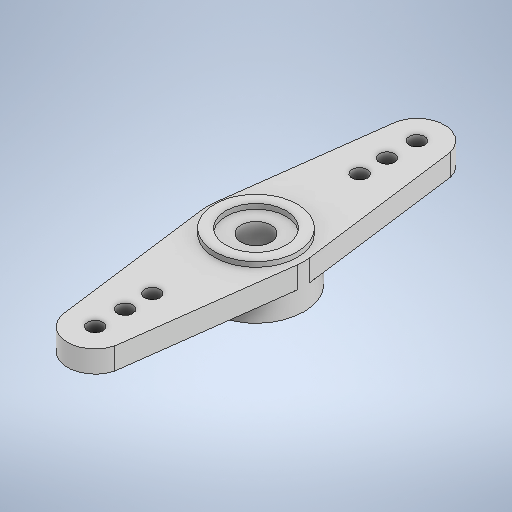
# Autodesk Inventor part: MMAE 232 Assignment 2_White Propellor - Dylan Tamras
Saved by Autodesk Inventor 2025.2 (Build 292293000, 293)
## iProperties
Created: 2025-01-19
Part Number: MMAE 232 Assignment 2_White Propellor - Dylan Tamras
Material: Generic
Document SubType Name: Modeling
Designer: Dylan
Density: 1 g/cm^3
Appearance: Default
Author: VRK99-0110
Title: Servo - White Propellor
Autodesk Inventor part; units mm, degrees
ref_plane "YZ Plane" through (0, 0, 0) normal (1, 0, 0) x (0, 1, 0)
ref_plane "XZ Plane" through (0, 0, 0) normal (0, 1, 0) x (-1, 0, 0)
ref_plane "XY Plane" through (0, 0, 0) normal (0, 0, 1) x (1, 0, 0)
sketch "Sketch1" plane through (0, 0, 0) normal (0, 1, 0) x (-1, 0, 0)
  line L0 (0, 0) -> (0, -14.74)
  arc A0 (-2.52, -14.74) -> (2.52, -14.74) centre (0, -14.74) ccw
  line L1 (2.4362, -15.3846) -> (4.3633, -0.5675)
  line L2 (-4.3633, -0.5675) -> (-2.4362, -15.3846)
  line L3 (0, 0) -> (0, 14.74)
  arc A1 (2.52, 14.74) -> (-2.52, 14.74) centre (0, 14.74) ccw
  circle A2 centre (0, 0) radius 4.4
  line L4 (2.4362, 15.3846) -> (4.3633, 0.5675)
  line L5 (-4.3633, 0.5675) -> (-2.4362, 15.3846)
  point P0 (4.3633, -0.5675)
  dimension "d2" = 2.52
  constraints: 12 end point, 10 point on circle, 3 centre point, 2 coincident, 1 vertical
  measures "d2" radius of A0
extrude "Extrusion1" add sketch "Sketch1" along normal blind 2 contours L3 A2 L0 | L0 A2 L3 | A2 L1 A0 L2 | A2 L5 A1 L4
sketch "Sketch2" plane through (0, 2, 0) normal (0, 1, 0) x (1, 0, 0)
  circle A0 centre (0, 14.74) radius 0.7
  circle A1 centre (0, 12) radius 0.7
  circle A2 centre (0, 9.5) radius 0.7
  circle A3 centre (0, -14.74) radius 0.7
  circle A4 centre (0, -12) radius 0.7
  circle A5 centre (0, -9.5) radius 0.7
  point P0 (0, 0)
  dimension "d7" = 1.4
  dimension "d9" = 1.4
  dimension "d11" = 1.4
  constraints: 6 centre point
  measures "d7" diameter of A0
  measures "d9" diameter of A1
  measures "d11" diameter of A2
extrude "Extrusion2" cut sketch "Sketch2" against normal blind 2
sketch "Sketch3" plane through (0, 2, 0) normal (0, 1, 0) x (1, 0, 0)
  circle A0 centre (0, 0) radius 1.375
  dimension "d14" = 2.75
  constraints: 1 centre point, 1 coincident
  measures "d14" diameter of A0
extrude "Extrusion3" cut sketch "Sketch3" against normal blind 2
sketch "Sketch4" plane through (0, 2, 0) normal (0, 1, 0) x (1, 0, 0)
  circle A0 centre (0, 0) radius 2.75
  circle A1 centre (0, 0) radius 3.785
  dimension "d18" = 5.5
  dimension "d19" = 7.57
  constraints: 2 centre point, 2 coincident
  measures "d18" diameter of A0
  measures "d19" diameter of A1
extrude "Extrusion4" add sketch "Sketch4" along normal blind 0.45
sketch "Sketch5" plane through (0, 0, 0) normal (0, -1, 0) x (1, 0, 0)
  circle A0 centre (0, 0) radius 4.4
  dimension "d22" = 8.8
  constraints: 1 centre point, 1 coincident
  measures "d22" diameter of A0
extrude "Extrusion5" add sketch "Sketch5" along normal blind 2
sketch "Sketch6" plane through (0, -2, 0) normal (0, -1, 0) x (1, 0, 0)
  circle A0 centre (0, 0) radius 1.375
  dimension "d25" = 2.75
  constraints: 1 centre point, 1 coincident
  measures "d25" diameter of A0
extrude "Extrusion6" cut sketch "Sketch6" against normal blind 2
body "Solid1"
